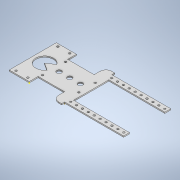
# Autodesk Inventor part: Frame
Saved by Autodesk Inventor 2022 (Build 260153000, 153)
## iProperties
Created: 2022-10-10
Part Number: Frame
Material: Generic
Document SubType Name: Modeling
Designer: Kilian De Ruyck
Density: 1 g/cm^3
Appearance: Default
Author: Kilian De Ruyck
Autodesk Inventor part; units mm, degrees
ref_plane "YZ Plane" through (0, 0, 0) normal (1, 0, 0) x (0, 1, 0)
ref_plane "XZ Plane" through (0, 0, 0) normal (0, 1, 0) x (-1, 0, 0)
ref_plane "XY Plane" through (0, 0, 0) normal (0, 0, 1) x (1, 0, 0)
sketch "Sketch23" plane through (0, 0, 0) normal (0, 1, 0) x (-1, 0, 0)
  line L0 (0, 0) -> (-100, 0)
  line L1 (-100, 0) -> (-100, -10)
  line L2 (-100, -10) -> (0, -10)
  line L3 (0, -10) -> (0, 0)
  line L4 (0, -10) -> (0, -70)
  line L5 (0, -70) -> (-100, -70)
  line L6 (-100, -70) -> (-100, -80)
  line L7 (-100, -80) -> (0, -80)
  line L8 (0, -80) -> (0, -70)
  dimension "d242" = 100
  dimension "d243" = 10
  dimension "d244" = 60
  dimension "d245" = 100
  dimension "d246" = 10
  constraints: 18 end point, 4 parallel, 2 horizontal, 2 perpendicular, 1 vertical
  measures "d242" distance of L2.end L1.end
  measures "d243" distance of L1.end L0.end
  measures "d244" distance of L2.end L4.end
  measures "d245" distance of L7.end L6.end
  measures "d246" distance of L6.end L5.end
extrude "Extrusion14" add sketch "Sketch23" along normal blind 2
sketch "Sketch24" plane through (0, 2, 0) normal (0, 1, 0) x (1, 0, 0)
  line L0 (0, 10) -> (0, 0) projected
  line L1 (0, 0) -> (-96, 0)
  line L2 (-96, 0) -> (-96, 80)
  line L3 (-96, 80) -> (0, 80)
  line L4 (0, 80) -> (0, 0)
  dimension "d249" = 96
  dimension "d250" = 80
  constraints: 8 end point, 2 parallel, 1 horizontal, 1 perpendicular
  measures "d249" distance of L2.end L3.end
  measures "d250" distance of L1.end L2.end
extrude "Extrusion15" add sketch "Sketch24" against normal blind 2
sketch "Sketch27" plane through (0, 2, 0) normal (0, 1, 0) x (1, 0, 0)
  line L0 (-96, 80) -> (-96, 0) projected
  line L1 (-96, 0) -> (100, 0) projected
  line L2 (0, 10) -> (0, 70) projected
  point P0 (0, 0)
  point P1 (-58, 20.5)
  point P2 (-58, 59.5)
  point P3 (-2, 26)
  point P4 (-2, 54)
  dimension "d253" = 39
  dimension "d254" = 28
  dimension "d255" = 5.5
  dimension "d256" = 5.5
  dimension "d257" = 0
  dimension "d259" = 20.5
  dimension "d269" = 56
  dimension "d270" = 38
  measures "d253" distance of point (-58, 59.5) point (-58, 20.5)
  measures "d254" distance of point (-2, 54) point (-2, 26)
  measures "d255" vertical distance of point (-58, 20.5) point (-2, 26)
  measures "d256" vertical distance of point (-58, 59.5) point (-2, 54)
  measures "d257" horizontal distance of point (-2, 26) point (-2, 54)
  measures "d259" distance from line of L1 point (-58, 20.5)
  measures "d269" horizontal distance of point (-2, 26) point (-58, 20.5)
  measures "d270" distance from line of L0 point (-58, 20.5)
hole "Hole8" at (-58, 2, -20.5) at (-58, 2, -59.5) at (-2, 2, -54) at (-2, 2, -26) direction (0, -1, 0) diameter 3.5 depth 2
sketch "Sketch28" plane through (0, 2, 0) normal (0, 1, 0) x (1, 0, 0)
  line L0 (0, 0) -> (-96, 0)
  line L1 (-96, 0) -> (-96, -5)
  line L2 (-96, -5) -> (0, -5)
  line L3 (0, -5) -> (0, 0)
  line L4 (100, 80) -> (-96, 80) projected
  line L5 (0, 80) -> (-96, 80)
  line L6 (-96, 80) -> (-96, 85)
  line L7 (-96, 85) -> (0, 85)
  line L8 (0, 85) -> (0, 80)
  dimension "d271" = 5
  dimension "d272" = 5
  constraints: 16 end point, 4 parallel, 3 point on line, 2 horizontal, 2 perpendicular
  measures "d271" distance of L1.end L0.end
  measures "d272" distance of L5.end L6.end
extrude "Extrusion16" add sketch "Sketch28" against normal blind 2
sketch "Sketch29" plane through (0, 2, 0) normal (0, 1, 0) x (1, 0, 0)
  line L0 (0, 0) -> (0, -5) projected
  line L1 (0, -5) -> (-15, -5)
  line L2 (0, -5) -> (-96, -5) projected
  line L3 (-15, -5) -> (-60, -5)
  line L4 (-60, -5) -> (-60, 15)
  line L5 (-60, 15) -> (-15, 15)
  line L6 (-15, 15) -> (-15, -5)
  line L7 (0, 85) -> (-15, 85)
  line L8 (-96, 85) -> (0, 85) projected
  line L9 (-15, 85) -> (-60, 85)
  line L10 (-60, 85) -> (-60, 65)
  line L11 (-60, 65) -> (-15, 65)
  line L12 (-15, 65) -> (-15, 85)
  point P0 (-60, 85)
  dimension "d275" = 15
  dimension "d276" = 45
  dimension "d277" = 20
  dimension "d278" = 15
  dimension "d279" = 45
  dimension "d280" = 20
  constraints: 20 end point, 4 parallel, 2 horizontal, 2 perpendicular, 2 point on line
  measures "d275" distance of L0.end L1.end
  measures "d276" distance of L4.end L5.end
  measures "d277" distance of L3.end L4.end
  measures "d278" distance of L7.start L7.end
  measures "d279" distance of L11.end L10.end
  measures "d280" distance of L10.end L9.end
extrude "Extrusion17" cut sketch "Sketch29" against normal blind 2
sketch "Sketch31" plane through (0, 0, 0) normal (0, -1, 0) x (1, 0, 0)
  line L0 (0, -70) -> (0, -10) projected
  line L1 (0, 0) -> (100, 0) projected
  line L2 (0, -70) -> (100, -70) projected
  point P0 (5, -5.263)
  point P1 (15, -5.263)
  point P2 (25, -5.263)
  point P3 (35, -5.263)
  point P4 (45, -5.263)
  point P5 (55, -5.263)
  point P6 (65, -5.263)
  point P7 (75, -5.263)
  point P8 (85, -5.263)
  point P9 (95, -5.263)
  point P10 (5, -74.737)
  point P11 (15, -74.737)
  point P12 (25, -74.737)
  point P13 (35, -74.737)
  point P14 (45, -74.737)
  point P15 (55, -74.737)
  point P16 (65, -74.737)
  point P17 (75, -74.737)
  point P18 (85, -74.737)
  point P19 (95, -74.737)
  dimension "d298" = 5
  dimension "d299" = 5.263
  dimension "d300" = 5.263
  dimension "d301" = 5.263
  dimension "d302" = 5.263
  dimension "d303" = 5.263
  dimension "d304" = 5.263
  dimension "d305" = 10
  dimension "d306" = 10
  dimension "d307" = 10
  dimension "d308" = 10
  dimension "d309" = 10
  dimension "d310" = 5.263
  dimension "d311" = 10
  dimension "d312" = 5.263
  dimension "d313" = 10
  dimension "d314" = 5.263
  dimension "d315" = 10
  dimension "d316" = 5.263
  dimension "d317" = 10
  dimension "d318" = 4.737
  dimension "d319" = 5
  dimension "d320" = 4.737
  dimension "d321" = 4.737
  dimension "d322" = 4.737
  dimension "d323" = 4.737
  dimension "d324" = 4.737
  dimension "d325" = 4.737
  dimension "d326" = 4.737
  dimension "d327" = 4.737
  dimension "d328" = 4.737
  dimension "d329" = 10
  dimension "d330" = 10
  dimension "d331" = 10
  dimension "d332" = 10
  dimension "d333" = 10
  dimension "d334" = 10
  dimension "d335" = 10
  dimension "d336" = 10
  dimension "d337" = 10
  measures "d298" distance from line of L0 point (5, -5.263)
  measures "d299" distance from line of L1 point (5, -5.263)
  measures "d300" distance from line of L1 point (15, -5.263)
  measures "d301" distance from line of L1 point (25, -5.263)
  measures "d302" distance from line of L1 point (35, -5.263)
  measures "d303" distance from line of L1 point (45, -5.263)
  measures "d304" distance from line of L1 point (55, -5.263)
  measures "d305" distance of point (5, -5.263) point (15, -5.263)
  measures "d306" distance of point (15, -5.263) point (25, -5.263)
  measures "d307" distance of point (25, -5.263) point (35, -5.263)
  measures "d308" distance of point (35, -5.263) point (45, -5.263)
  measures "d309" distance of point (45, -5.263) point (55, -5.263)
  measures "d310" distance from line of L1 point (65, -5.263)
  measures "d311" distance of point (55, -5.263) point (65, -5.263)
  measures "d312" distance from line of L1 point (75, -5.263)
  measures "d313" distance of point (65, -5.263) point (75, -5.263)
  measures "d314" distance from line of L1 point (85, -5.263)
  measures "d315" distance of point (75, -5.263) point (85, -5.263)
  measures "d316" distance from line of L1 point (95, -5.263)
  measures "d317" distance of point (85, -5.263) point (95, -5.263)
  measures "d318" distance from line of L2 point (5, -74.737)
  measures "d319" distance from line of L0 point (5, -74.737)
  measures "d320" distance from line of L2 point (15, -74.737)
  measures "d321" distance from line of L2 point (25, -74.737)
  measures "d322" distance from line of L2 point (35, -74.737)
  measures "d323" distance from line of L2 point (45, -74.737)
  measures "d324" distance from line of L2 point (55, -74.737)
  measures "d325" distance from line of L2 point (65, -74.737)
  measures "d326" distance from line of L2 point (75, -74.737)
  measures "d327" distance from line of L2 point (85, -74.737)
  measures "d328" distance from line of L2 point (95, -74.737)
  measures "d329" distance of point (85, -74.737) point (95, -74.737)
  measures "d330" distance of point (75, -74.737) point (85, -74.737)
  measures "d331" distance of point (65, -74.737) point (75, -74.737)
  measures "d332" distance of point (55, -74.737) point (65, -74.737)
  measures "d333" distance of point (45, -74.737) point (55, -74.737)
  measures "d334" distance of point (45, -74.737) point (35, -74.737)
  measures "d335" distance of point (25, -74.737) point (35, -74.737)
  measures "d336" distance of point (15, -74.737) point (25, -74.737)
  measures "d337" distance of point (5, -74.737) point (15, -74.737)
hole "Hole10" at (5, 0, -5.263) at (15, 0, -5.263) at (25, 0, -5.263) at (35, 0, -5.263) at (45, 0, -5.263) at (55, 0, -5.263) at (65, 0, -5.263) at (75, 0, -5.263) at (85, 0, -5.263) at (95, 0, -5.263) at (5, 0, -74.737) at (15, 0, -74.737) at (25, 0, -74.737) at (35, 0, -74.737) at (45, 0, -74.737) at (55, 0, -74.737) at (65, 0, -74.737) at (75, 0, -74.737) at (85, 0, -74.737) at (95, 0, -74.737) direction (0, 1, 0) diameter 3.5 depth 2
sketch "Sketch32" plane through (0, 0, 0) normal (0, -1, 0) x (1, 0, 0)
  line L0 (-96, 5) -> (-60, 5) projected
  line L1 (-60, -85) -> (-96, -85) projected
  line L2 (-96, 5) -> (-94, 5)
  line L3 (-94, 5) -> (-94, -85)
  line L4 (-94, -85) -> (-96, -85)
  line L5 (-96, -85) -> (-96, 5)
  point P0 (0, 0)
  dimension "d345" = 2
  constraints: 8 end point, 2 parallel, 1 horizontal, 1 perpendicular, 1 point on line
  measures "d345" distance of L3.end L4.end
extrude "Extrusion18" cut sketch "Sketch32" against normal blind 2
fillet "Fillet6" radius 10 2 edges at (-15, 1, -85) (-15, 1, 5)
sketch "Sketch34" plane through (-60, 2, 5) normal (1, 0, 0) x (0, 0, -1)
  point P0 (5, -2)
sketch "Sketch35" plane through (0, 2, 0) normal (0, 1, 0) x (1, 0, 0)
  line L0 (-94, -5) -> (-60, -5) projected
  line L1 (-60, -5) -> (-94, -5)
  line L2 (-94, -5) -> (-94, 0)
  line L3 (-94, 0) -> (-60, 0)
  line L4 (-60, 0) -> (-60, -5)
  line L5 (-94, 85) -> (-94, -5) projected
  line L6 (-60, 65) -> (-60, 85) projected
  line L7 (-94, 85) -> (-60, 85)
  line L8 (-60, 85) -> (-60, 80)
  line L9 (-60, 80) -> (-94, 80)
  line L10 (-94, 80) -> (-94, 85)
  point P0 (0, 0)
  dimension "d354" = 5
  constraints: 16 end point, 4 parallel, 2 horizontal, 2 perpendicular, 1 point on line
  measures "d354" distance of L7.end L8.end
extrude "Extrusion20" cut sketch "Sketch35" against normal blind 10
sketch "Sketch36" plane through (0, 2, 0) normal (0, 1, 0) x (1, 0, 0)
  line L0 (-60, 80) -> (-94, 80) projected
  line L1 (-94, 0) -> (-60, 0) projected
  line L2 (-94, 0) -> (-60, 0) projected
  line L3 (-60, 0) -> (-60, 15) projected
  line L4 (-94, 80) -> (-94, 0) projected
  point P0 (0, 0)
  point P1 (-87, 4.5)
  point P2 (-67, 4.5)
  point P3 (-87, 75.5)
  point P4 (-67, 75.5)
  point P5 (-67.6771, 80)
  point P6 (-84.3229, 80)
  point P7 (-87.6771, 0)
  point P8 (-84.3229, 0)
  point P9 (-67.6771, 0)
  dimension "d357" = 4.5
  dimension "d358" = 4.5
  dimension "d359" = 4.5
  dimension "d360" = 4.5
  dimension "d361" = 20
  dimension "d362" = 7
  dimension "d363" = 7
  dimension "d364" = 20
  measures "d357" distance from line of L0 point (-87, 75.5)
  measures "d358" distance from line of L0 point (-67, 75.5)
  measures "d359" distance from line of L1 point (-87, 4.5)
  measures "d360" distance from line of L2 point (-67, 4.5)
  measures "d361" distance of point (-67, 4.5) point (-87, 4.5)
  measures "d362" distance from line of L3 point (-67, 4.5)
  measures "d363" distance from line of L4 point (-87, 75.5)
  measures "d364" distance of point (-87, 75.5) point (-67, 75.5)
hole "Hole11" at (-87, 2, -4.5) at (-67, 2, -4.5) at (-87, 2, -75.5) at (-67, 2, -75.5) direction (0, -1, 0) diameter 3.5 depth 2
sketch "Sketch37" plane through (0, 2, 0) normal (0, 1, 0) x (1, 0, 0)
  line L0 (100, 10) -> (0, 10) projected
  line L1 (0, 70) -> (5, 70)
  line L2 (5, 70) -> (5, 10)
  line L3 (5, 10) -> (0, 10)
  line L4 (0, 10) -> (0, 70)
  point P0 (0, 0)
  dimension "d372" = 5
  constraints: 8 end point, 2 parallel, 1 horizontal, 1 perpendicular, 1 point on line
  measures "d372" distance of L2.end L3.end
extrude "Extrusion21" add sketch "Sketch37" against normal blind 2
sketch "Sketch38" plane through (0, 2, 0) normal (0, 1, 0) x (1, 0, 0)
  circle A0 centre (-74, 40) radius 15
  line L0 (-94, 80) -> (-94, 0) projected
  line L1 (-94, 0) -> (-60, 0) projected
  point P0 (0, 0)
  dimension "d375" = 30
  dimension "d376" = 20
  dimension "d377" = 40
  constraints: 1 centre point
  measures "d375" diameter of A0
  measures "d376" distance from line of L0 A0.centre
  measures "d377" distance from line of L1 A0.centre
extrude "Extrusion22" cut sketch "Sketch38" against normal blind 2
sketch "Sketch39" plane through (0, 2, 0) normal (0, 1, 0) x (1, 0, 0)
  circle A0 centre (-74, 40) radius 15 projected
  circle A1 centre (-34, 40) radius 5 projected
  line L0 (-59, 40) -> (-59, 50)
  line L1 (-59, 50) -> (-59, 30)
  line L2 (-74, 40) -> (-59, 50)
  line L3 (-74, 40) -> (-59, 30)
  point P0 (0, 0)
  point P1 (-61.5192, 31.6795)
  point P2 (-61.5192, 48.3205)
  dimension "d380" = 10
  dimension "d381" = 20
  constraints: 8 end point, 1 point on line, 2 other
  measures "d380" distance of L0.start L0.end
  measures "d381" distance of L0.end L1.end
extrude "Extrusion23" add sketch "Sketch39" against normal blind 2 contours A0 L3 L2 picked at (-64.475, 37.1161)
sketch "Sketch40" plane through (0, 2, 0) normal (0, 1, 0) x (1, 0, 0)
  circle A0 centre (-49, 39.6429) radius 4
  circle A1 centre (-13, 39.6429) radius 4
  circle A2 centre (-31, 39.6429) radius 4
  line L0 (-94, 80) -> (-94, 0) projected
  point P0 (0, 0)
  dimension "d384" = 8
  dimension "d385" = 8
  dimension "d386" = 8
  dimension "d387" = 45
  dimension "d388" = 18
  dimension "d389" = 18
  constraints: 3 centre point
  measures "d384" diameter of A0
  measures "d385" diameter of A1
  measures "d386" diameter of A2
  measures "d387" distance from line of L0 A0.centre
  measures "d388" distance of A0.centre A2.centre
  measures "d389" distance of A2.centre A1.centre
extrude "Extrusion24" cut sketch "Sketch40" against normal blind 2
equation "\"d300\" = d299"
equation "\"d301\" = d300"
equation "\"d302\" = d301"
equation "\"d303\" = d302"
equation "\"d304\" = d303"
equation "\"d310\" = d304"
equation "\"d312\" = d310"
equation "\"d314\" = d312"
equation "\"d316\" = d314"
equation "\"d320\" = d318"
equation "\"d321\" = d320"
equation "\"d322\" = d321"
equation "\"d323\" = d322"
equation "\"d324\" = d323"
equation "\"d325\" = d324"
equation "\"d326\" = d325"
equation "\"d327\" = d326"
equation "\"d328\" = d327"
body "Solid3"
